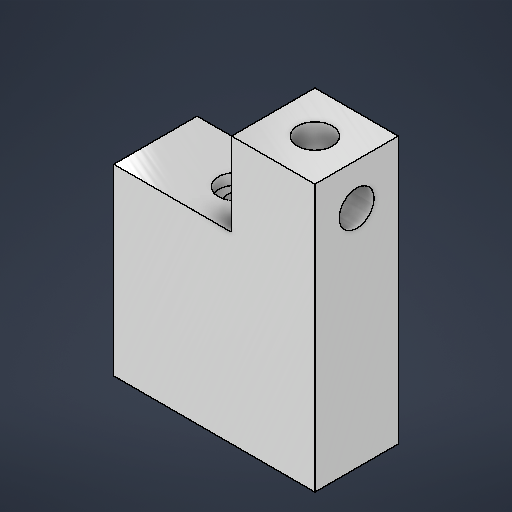
# Autodesk Inventor part: B Idler (Tulip)
Saved by Autodesk Inventor 2026 (Build 300175050, 175E)
## iProperties
Created: 2025-04-15
Part Number: B Idler (Tulip)
Material: Aluminum 6061
Document SubType Name: Modeling
Designer: Joshua Eah
Density: 2.7 g/cm^3
Appearance: Aluminum - Flat
Author: Joshua Eah
Autodesk Inventor part; units mm, degrees
ref_plane "YZ Plane" through (0, 0, 0) normal (1, 0, 0) x (0, 1, 0)
ref_plane "XZ Plane" through (0, 0, 0) normal (0, 1, 0) x (-1, 0, 0)
ref_plane "XY Plane" through (0, 0, 0) normal (0, 0, 1) x (1, 0, 0)
sketch "Sketch1" plane through (0, 0, 0) normal (0, 1, 0) x (-1, 0, 0)
  line L0 (0, 0) -> (36.2103, 0)
  line L1 (36.2103, 0) -> (36.2103, -15)
  line L2 (36.2103, -15) -> (0, -15)
  line L3 (0, -15) -> (0, 0)
  dimension "d0" = 36.2103
  dimension "d1" = 15
  constraints: 8 end point, 2 parallel, 1 horizontal, 1 perpendicular
  measures "d0" distance of L1.end L2.end
  measures "d1" distance of L0.end L1.end
extrude "Extrusion1" add sketch "Sketch1" along normal blind 48
sketch "Sketch5" plane through (0, 48, 0) normal (0, 1, 0) x (1, 0, 0)
  line L0 (0, 15) -> (-36.2103, 15) projected
  line L1 (-36.2103, 15) -> (-36.2103, 0) projected
  line L2 (-36.2103, 0) -> (0, 0) projected
  line L3 (0, 0) -> (0, 15) projected
  line L4 (-36.2103, 0) -> (0, 0) projected
  line L5 (0, 0) -> (-15, 0)
  line L6 (-15, 0) -> (-15, 15)
  line L7 (-15, 15) -> (0, 15)
  line L8 (0, 15) -> (0, 0)
  dimension "d72" = 15
  constraints: 8 end point, 2 parallel, 1 horizontal, 1 perpendicular, 1 point on line
  measures "d72" distance of L6.end L7.end
extrude "Extrusion5" cut sketch "Sketch5" against normal blind 15 contours L6 L2 L1 L0
sketch "Sketch6" plane through (0, 33, 0) normal (0, 1, 0) x (1, 0, 0)
  line L0 (-36.2103, 15) -> (-15, 15) projected
  line L1 (-36.2103, 0) -> (-36.2103, 15) projected
  line L2 (-15, 0) -> (-36.2103, 0) projected
  circle A0 centre (-21.7, 7.5) radius 1.3741
  line L3 (0, 0) -> (0, 15) projected
  line L4 (-15, 15) -> (-15, 0) projected
  dimension "d23" = 7.5
  dimension "d24" = 21.7
  constraints: 1 centre point
  measures "d23" distance from line of A0.centre L2
  measures "d24" distance from line of L3 A0.centre
hole "Hole1" at (-21.7, 33, -7.5) direction (0, -1, 0) diameter 3.2004 end through all counterbore diameter 6.2992 counterbore depth 2 clearance for "Oval Head Machine Screw" size "M3" standard "Ansi Metric M Profile"
sketch "Sketch7" plane through (0, 48, 0) normal (0, 1, 0) x (1, 0, 0)
  line L0 (-15, 0) -> (0, 0) projected
  line L1 (0, 0) -> (0, 15) projected
  line L2 (0, 15) -> (-15, 15) projected
  circle A0 centre (-7.5, 7.5) radius 1.6
  line L3 (-15, 15) -> (-15, 0) projected
  dimension "d32" = 3.2
  dimension "d33" = 7.5
  dimension "d34" = 7.5
  constraints: 1 centre point
  measures "d32" diameter of A0
  measures "d33" distance from line of L0 A0.centre
  measures "d34" distance from line of L1 A0.centre
hole "Hole2" at (-7.5, 48, -7.5) direction (0, -1, 0) diameter 3.2004 end through all counterbore diameter 6.2992 counterbore depth 17 clearance for "Oval Head Machine Screw" size "M3" standard "Ansi Metric M Profile"
sketch "Sketch8" plane through (0, 48, 0) normal (1, 0, 0) x (0, 0, -1)
  line L0 (15, -48) -> (15, 0) projected
  line L1 (0, 0) -> (15, 0) projected
  line L2 (0, -48) -> (0, 0) projected
  circle A0 centre (7.5, -7.5) radius 1.6
  line L3 (0, -48) -> (15, -48) projected
  dimension "d42" = 3.2
  dimension "d43" = 7.5
  dimension "d44" = 7.5
  constraints: 1 centre point
  measures "d42" diameter of A0
  measures "d43" distance from line of L1 A0.centre
  measures "d44" distance from line of L2 A0.centre
hole "Hole3" at (0, 40.5, -7.5) direction (-1, 0, 0) diameter 3.2004 end through all counterbore diameter 6.2992 counterbore depth 12 clearance for "Oval Head Machine Screw" size "M3" standard "Ansi Metric M Profile"
body "Solid1"
